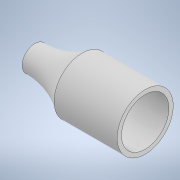
# Autodesk Inventor part: 5 mm nozle
Saved by Autodesk Inventor 2022 (Build 260153000, 153)
## iProperties
Created: 2023-01-19
Part Number: 5 mm nozle
Material: Generic
Document SubType Name: Modeling
Designer: ASUS
Density: 1 g/cm^3
Appearance: Default
Author: ASUS
Autodesk Inventor part; units mm, degrees
ref_plane "YZ Plane" through (0, 0, 0) normal (1, 0, 0) x (0, 1, 0)
ref_plane "XZ Plane" through (0, 0, 0) normal (0, 1, 0) x (-1, 0, 0)
ref_plane "XY Plane" through (0, 0, 0) normal (0, 0, 1) x (1, 0, 0)
sketch "Sketch1" plane through (0, 0, 0) normal (1, 0, 0) x (0, 1, 0)
  circle A0 centre (0, 0) radius 7.5
  circle A1 centre (0, 0) radius 8.875
  dimension "d0" = 15
  dimension "d1" = 17.75
  constraints: 2 centre point, 2 coincident
  measures "d0" diameter of A0
  measures "d1" diameter of A1
extrude "Extrusion1" add sketch "Sketch1" along normal blind 20
sketch "Sketch2" plane through (0, 0, 0) normal (0, 0, 1) x (1, 0, 0)
  line L0 (-15, 0) -> (-15, 4) construction
  arc A0 (-15, 4) -> (0, 8.875) centre (-15, 29.5144) ccw
  line L1 (-15, 4) -> (-2.0685, 4) construction
  arc A1 (-13.9, 2.9227) -> (0, 7.5297) centre (-15, 29.5144) ccw
  line L2 (-13.9, 2.9227) -> (-13.9, 0) construction
  line L3 (0, -8.875) -> (0, 8.875) projected
  line L4 (0, 8.875) -> (0, 7.5297)
  line L5 (-13.9, 2.9227) -> (-15, 2.9227)
  line L6 (-15, 2.9227) -> (-15, 4)
  line L7 (0, 0) -> (-13.9, 0) construction
  dimension "d4" = 15
  dimension "d6" = 4
  dimension "d7" = 1.1
  constraints: 14 end point, 4 point on circle, 2 centre point, 2 horizontal, 2 point on line, 1 collinear, 1 perpendicular, 1 tangent, 1 vertical
  measures "d4" distance of L7.start L0.start
  measures "d6" distance of L0.start L0.end
  measures "d7" radial gap between concentric circles of A0 A1
revolve "Revolution1" add sketch "Sketch2" angle 360 about axis through (0, 0, 0) along (-1, 0, 0)
body "Solid1"
